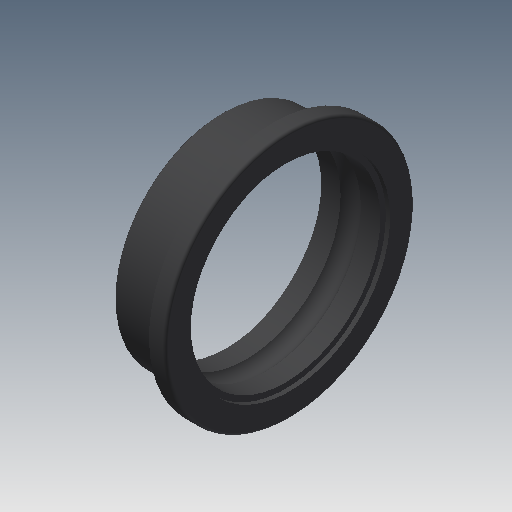
# Autodesk Inventor part: MF85ZZ Outer Ring
Saved by Autodesk Inventor 2017.3 (Build 213256000, 256)
## iProperties
Category: PARTsolutions
Company: NSK_RB
Created: 2016-04-26
Part Number: MF85ZZ Outer Ring
Catalog Web Link: www.cadenas.de
Description: shielded_type_zz_zzs_OR-
Vendor: NSK_RB
Document SubType Name: Modeling
Designer: psAdmin
Manufacturer: NSK_RB
Mass: 0.0352807 g
Surface Area: 1.77822 cm^2
Volume: 0.0352807 cm^3
Density: 1 g/cm^3
Material: 一般
Appearance: PSOLRGB-128-128-128
PSOL_IDENT_0: {$CADENAS_DATA\23d-libs\nsk_rb\roller_bearings\deep_groove_bb\exstra_small_miniatur_bb\metric_design
PSOL_IDENT_1: _with_flange\shielded_type_zz_zzs_or1.prj},194 {VTYP=3D},{NB=MF85ZZ Outer Ring},{LINA=MF85ZZ Outer R
PSOL_IDENT_2: ing},{NN=shielded_type_zz_zzs_OR},{DATE=18.06.2013 02:54:38},{GEOMDATE=04.01.2008 00:00:00},{VERSION=
PSOL_IDENT_3: },{LINEID=210},{LINESUBID=-1},{WBVAR=}  {NB=MF85ZZ Outer Ring},{LINA=MF85ZZ Outer Ring},{KT=DUMMY},{
PSOL_IDENT_4: IDNR=},{STAN=},{ORDER=MF85ZZ},{SD=5.0},{X=5.0},{D=8},{DD=8},{DD1=0.0},{D2=9.2},{DD2=9.2},{B=0.0},{B1=
PSOL_IDENT_5: 2.5},{CC1=0.0},{C2=0.6},{CC2=0.6},{R=0.00},{R1=0.10},{DI1=5.80},{DI2=5.80},{SDE1=7.00},{SDE2=7.40},{
PSOL_IDENT_6: CR1=310},{COR1=120},{CR2=31},{COR2=12.0},{LG=53000},{LO=63000},{DA=0.0},{DB=5.8},{RA=0.00},{RB=0.10}
PSOL_IDENT_7: ,{MASS=0.41},{SC=1}
NN: shielded_type_zz_zzs_OR
NB: MF85ZZ Outer Ring
NBSYN: $ORDER. Outer Ring
LINA: MF85ZZ Outer Ring
ORDER: MF85ZZ
SD: 5.0
X: 5.0
D: 8
DD: 8
DD1: 0.0
D2: 9.2
DD2: 9.2
B: 0.0
B1: 2.5
CC1: 0.0
C2: 0.6
CC2: 0.6
R: 0.00
R1: 0.10
DI1: 5.80
DI2: 5.80
SDE1: 7.00
SDE2: 7.40
CR1: 310
COR1: 120
CR2: 31
COR2: 12.0
LG: 53000
LO: 63000
DA: 0.0
DB: 5.8
RA: 0.00
RB: 0.10
MASS: 0.41
SC: 1
SUPPLIER: NSK_RB
ARTICLENO: MF85ZZ Outer Ring
BOMINFO: MF85ZZ Outer Ring
CREATOR: CADENAS GmbH
Title: MF85ZZ Outer Ring
Author: Cadenas PARTsolutions
Autodesk Inventor part; units mm, degrees
sketch "Sketch_1" plane through (0, 0, 0) normal (0, 0, 1) x (1, 0, 0)
  line L0 (2.5, 0) -> (0, 0)
  line L1 (0, 3.7) -> (0.1562, 3.7)
  line L2 (0.1562, 3.7) -> (0.1562, 3.5)
  line L3 (0.1562, 3.5) -> (0.8758, 3.5)
  arc A0 (1.6242, 3.5) -> (0.8758, 3.5) centre (1.25, 3.25) ccw
  line L4 (1.6242, 3.5) -> (2.3438, 3.5)
  line L5 (2.3438, 3.5) -> (2.3438, 3.7)
  line L6 (2.3438, 3.7) -> (2.5, 3.7)
  line L7 (2.5, 3.7) -> (2.5, 4.5)
  arc A1 (2.5, 4.5) -> (2.4, 4.6) centre (2.4, 4.5) ccw
  line L8 (2.4, 4.6) -> (1.9, 4.6)
  line L9 (1.9, 4.6) -> (1.9, 4)
  line L10 (1.9, 4) -> (0.1, 4)
  arc A2 (0.1, 4) -> (0, 3.9) centre (0.1, 3.9) ccw
  line L11 (0, 3.9) -> (0, 3.7)
  constraints: 24 end point, 6 point on circle, 3 centre point
revolve "Revolution1" add sketch "Sketch_1" angle 360 about axis through (2.5, 0, 0) along (1, 0, 0)
ref_plane "ip_st_1_XY" through (0, 0, 0) normal (1, 0, 0) x (0, 0, -1)
ref_plane "ip_st_1_YZ" through (0, 0, 0) normal (0, 0, -1) x (0, 1, 0)
ref_plane "ip_st_1_ZX" through (0, 0, 0) normal (0, 1, 0) x (1, 0, 0)
ref_plane "ip_st_2_XY" through (2.3438, 0, 0) normal (-1, 0, 0) x (0, 0, -1)
ref_plane "ip_st_2_YZ" through (2.3438, 0, 0) normal (0, 0, -1) x (0, -1, 0)
ref_plane "ip_st_2_ZX" through (2.3438, 0, 0) normal (0, -1, 0) x (-1, 0, 0)
body "Solid1"
